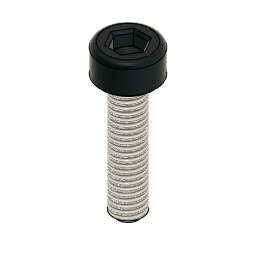
Breakout Box (Autodesk Fusion 360 archive; units mm, degrees)
design "Cap Head Screw M3x12"
part number: HW1292SC
Autodesk Fusion 360 part; units mm, degrees
sketch "Sketch1" plane through (0, 0, 0) normal (0, 0, 1) x (1, 0, 0)
  circle A0 centre (0, 0) radius 2.75
  line L0 (-0.7217, 1.25) -> (-1.4434, 0)
  line L1 (-1.4434, 0) -> (-0.7217, -1.25)
  line L2 (-0.7217, -1.25) -> (0.7217, -1.25)
  line L3 (0.7217, -1.25) -> (1.4434, 0)
  line L4 (1.4434, 0) -> (0.7217, 1.25)
  line L5 (0.7217, 1.25) -> (-0.7217, 1.25)
  circle A1 centre (0, 0) radius 1.5
  dimension "d5" = 5.5
  dimension "d6" = 1.25
  dimension "d12" = 3
  constraint coincident A0.centre A1.centre
  measures "d5" diameter of A0
  measures "d6" distance of A0.centre L5
  measures "d12" diameter of A1
extrude "Extrude1" add sketch "Sketch1" along normal blind 3 contours A0 | L0 L1 L2 L3 L4 L5 | A1
extrude "Extrude2" add sketch "Sketch1" along normal blind 0.75 contours L0 L1 L2 L3 L4 L5
hole "Hole1" at (0, 0, 3) direction (0, 0, -1) diameter 2.5 depth 1.3 tip angle 120
extrude "Extrude3" add sketch "Sketch1" against normal blind 12 contours L0 L1 L2 L3 L4 L5 | A1
extrude "Extrude4" cut sketch "Sketch1" against normal blind 1.3 from surface at 3 contours L0 L1 L2 L3 L4 L5
fillet "Fillet1" radius 0.5 1 edges at (-2.5639, -0.9944, 3)
fillet "Fillet2" radius 0.25 1 edges at (-1.3985, -0.5424, 0)
chamfer "Chamfer1" distance 0.25 angle 45 7 edges at (-1.0825, 0.625, 3) (-1.0825, -0.625, 3) (0, -1.25, 3) (1.0825, -0.625, 3) (1.0825, 0.625, 3) (0, 1.25, 3) (-2.5639, -0.9944, 0) tangent chain off
chamfer "Chamfer2" distance 0.5 angle 45 1 edges at (-1.3985, 0.5424, -12)
thread "Thread1" "ISO Metric profile 3.0 M3x0.5 6g" major diameter 2.927 minor diameter 2.3555 pitch 0.5 angle 60 resizes the face on face at (1.4925, -0.1494, -4)
equation "Thread_Size = 3 mm"
equation "Thread_Length = 12 mm"
equation "Head_Diameter = 5.5 mm"
equation "Hex_Width = 2.5 mm"
equation "d5 = Head_Diameter"
equation "d6 = Hex_Width / 2"
equation "Head_Height = 3 mm"
equation "d8 = Head_Height"
equation "d10 = Head_Height * 0.25"
equation "d12 = Thread_Size"
equation "d13 = -Thread_Length"
equation "d19 = Hex_Depth"
equation "d20 = Hex_Width"
equation "Hex_Depth = 1.3 mm"
equation "d24 = -Hex_Depth"
